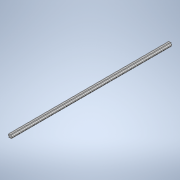
# Autodesk Inventor part: Churro 4in
Saved by Autodesk Inventor 2020 (Build 240168000, 168)
## iProperties
Created: 2020-01-14
Part Number: Churro 4in
Material: Generic
Document SubType Name: Modeling
Designer: aidan
Density: 1 g/cm^3
Appearance: Default
Author: aidan
Autodesk Inventor part; units mm, degrees
ref_plane "YZ Plane" through (0, 0, 0) normal (1, 0, 0) x (0, 1, 0)
ref_plane "XZ Plane" through (0, 0, 0) normal (0, 1, 0) x (-1, 0, 0)
ref_plane "XY Plane" through (0, 0, 0) normal (0, 0, 1) x (1, 0, 0)
sketch "Sketch1" plane through (0, 0, 0) normal (0, 0, 1) x (1, 0, 0)
  circle A0 centre (-4.8443, 5.8204) radius 6.35 construction
  arc A1 (-6.7493, 12.1704) -> (-2.9393, 12.1704) centre (-4.8443, 12.3033) ccw
  line L0 (-8.5105, 12.1704) -> (-6.7493, 12.1704)
  line L1 (-2.9393, 12.1704) -> (-1.1781, 12.1704)
  arc A2 (-0.2975, 10.6452) -> (1.6075, 7.3457) centre (0.7701, 9.0619) ccw
  arc A3 (1.6075, 4.2952) -> (-0.2975, 0.9957) centre (0.7701, 2.579) ccw
  arc A4 (-2.9393, -0.5296) -> (-6.7493, -0.5296) centre (-4.8443, -0.6625) ccw
  arc A5 (-9.3911, 0.9957) -> (-11.2961, 4.2952) centre (-10.4586, 2.579) ccw
  arc A6 (-11.2961, 7.3457) -> (-9.3911, 10.6452) centre (-10.4586, 9.0619) ccw
  line L2 (-12.1766, 5.8204) -> (-11.2961, 7.3457)
  line L3 (-8.5105, -0.5296) -> (-9.3911, 0.9957)
  line L4 (-1.1781, -0.5296) -> (-2.9393, -0.5296)
  line L5 (2.4881, 5.8204) -> (1.6075, 4.2952)
  line L6 (-1.1781, 12.1704) -> (-0.2975, 10.6452)
  line L7 (-9.3911, 10.6452) -> (-8.5105, 12.1704)
  line L8 (-11.2961, 4.2952) -> (-12.1766, 5.8204)
  line L9 (-6.7493, -0.5296) -> (-8.5105, -0.5296)
  line L10 (-0.2975, 0.9957) -> (-1.1781, -0.5296)
  line L11 (1.6075, 7.3457) -> (2.4881, 5.8204)
  point P0 (0, 0)
  point P1 (-4.8443, -0.5296)
  point P2 (-4.8443, 12.1704)
  point P3 (0.655, 8.9954)
  point P4 (0.655, 2.6454)
  point P5 (-4.8443, -0.5296)
  point P6 (-10.3436, 2.6454)
  point P7 (-10.3436, 8.9954)
  point P8 (-0.2975, 10.6452)
  point P9 (-9.3911, 10.6452)
  point P10 (-11.2961, 4.2952)
  point P11 (-9.3911, 0.9957)
  point P12 (-6.7493, -0.5296)
  point P13 (-2.9393, -0.5296)
  point P14 (1.6075, 7.3457)
  dimension "d2" = 12.7
  dimension "d7" = 360
  dimension "d11" = 360
  dimension "d15" = 360
  constraints: 24 end point, 12 point on circle, 6 centre point, 2 horizontal, 1 coincident, 1 vertical alignment, 73 other
extrude "Extrusion1" add sketch "Sketch1" along normal blind 558.8
sketch "Sketch2" plane through (0, 0, 558.8) normal (0, 0, 1) x (1, 0, 0)
  circle A0 centre (-4.8443, 5.8204) radius 2.9337
  line L0 (-8.5105, -0.5296) -> (-6.7493, -0.5296) projected
  line L1 (-8.5105, 12.1704) -> (-8.5105, -0.5296) construction
  line L2 (-1.1781, 12.1704) -> (-2.9393, 12.1704) projected
  line L3 (-2.9393, -0.5296) -> (-1.1781, -0.5296) projected
  line L4 (-1.1781, 12.1704) -> (-1.1781, -0.5296) construction
  line L5 (-4.8443, 9.4005) -> (-4.8443, 3.0295) construction
  point P0 (0, 0)
  dimension "d19" = 6.35
  dimension "d20" = 5.8674
  constraints: 6 end point, 3 vertical, 1 centre point, 1 point on line, 1 other
  measures "d19" distance from line of A0.centre L0
  measures "d20" diameter of A0
extrude "Extrusion2" cut sketch "Sketch2" against normal blind 558.8
equation "\"d17\" = d23"
equation "\"d21\" = d23"
equation "\"d23\" = 558.8"
body "Solid1"
